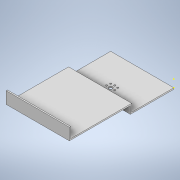
# Autodesk Inventor part: Single Sided board
Saved by Autodesk Inventor 2020.3 (Build 243373010, 373A)
## iProperties
Created: 2020-09-26
Part Number: Single Sided board
Material: Generic
Document SubType Name: Modeling
Designer: Owner
Density: 1 g/cm^3
Appearance: Default
Author: Owner
Autodesk Inventor part; units mm, degrees
ref_plane "YZ Plane" through (0, 0, 0) normal (1, 0, 0) x (0, 1, 0)
ref_plane "XZ Plane" through (0, 0, 0) normal (0, 1, 0) x (-1, 0, 0)
ref_plane "XY Plane" through (0, 0, 0) normal (0, 0, 1) x (1, 0, 0)
sketch "Sketch1" plane through (0, 0, 0) normal (0, 1, 0) x (-1, 0, 0)
  line L0 (0, 0) -> (152.4, 0)
  line L1 (152.4, 0) -> (152.4, 252.095)
  line L2 (152.4, 252.095) -> (0, 252.095)
  line L3 (0, 252.095) -> (0, 0)
  circle A0 centre (76.2, 76.2) radius 50.8
  circle A1 centre (76.2, 76.2) radius 4.5
  dimension "d0" = 152.4
  dimension "d1" = 252.095
  dimension "d2" = 101.6
  dimension "d3" = 9
  constraints: 8 end point, 2 centre point, 2 parallel, 1 coincident, 1 horizontal, 1 perpendicular
  measures "d0" distance of L2.end L1.end
  measures "d1" distance of L1.end L0.end
  measures "d2" diameter of A0
  measures "d3" diameter of A1
extrude "Extrusion1" add sketch "Sketch1" against normal blind 3.175 contours L3 L2 L1 L0 | A0
sketch "Sketch2" plane through (0, 0, 0) normal (0, 1, 0) x (1, 0, 0)
  line L0 (0, -252.095) -> (-152.4, -252.095) projected
  line L1 (-152.4, -252.095) -> (-152.4, 0) projected
  line L2 (0, -252.095) -> (-152.4, -252.095)
  line L3 (-152.4, -252.095) -> (-152.4, -248.92)
  line L4 (-152.4, -248.92) -> (0, -248.92)
  line L5 (0, -248.92) -> (0, -252.095)
  point P0 (0, 0)
  dimension "d6" = 3.175
  constraints: 8 end point, 2 parallel, 1 horizontal, 1 perpendicular, 1 point on line
  measures "d6" distance of L2.end L3.end
extrude "Extrusion2" add sketch "Sketch2" along normal blind 25.4
sketch "Sketch3" plane through (0, 0, 0) normal (0, 1, 0) x (1, 0, 0)
  circle A0 centre (-66.421, -76.2) radius 2
  circle A1 centre (-85.979, -76.2) radius 2
  circle A2 centre (-76.2, -66.421) radius 2
  circle A3 centre (-76.2, -85.979) radius 2
  point P0 (0, 0)
  dimension "d9" = 4
  dimension "d10" = 4
  dimension "d11" = 4
  dimension "d12" = 4
  constraints: 4 centre point
  measures "d9" diameter of A0
  measures "d10" diameter of A1
  measures "d11" diameter of A2
  measures "d12" diameter of A3
extrude "Extrusion3" cut sketch "Sketch3" against normal blind 25.4
sketch "Sketch4" plane through (0, 0, 0) normal (0, 1, 0) x (1, 0, 0)
  circle A0 centre (-76.2, -85.979) radius 2 projected
  circle A1 centre (-76.2, -85.979) radius 2
  circle A2 centre (-76.2, -76.2) radius 4.5 projected
  circle A3 centre (-76.2, -76.2) radius 4.5
  circle A4 centre (-83.1148, -83.1148) radius 2
  circle A5 centre (-76.2, -76.2) radius 4.5
  circle A6 centre (-85.979, -76.2) radius 2
  circle A7 centre (-76.2, -76.2) radius 4.5
  circle A8 centre (-83.1148, -69.2852) radius 2
  circle A9 centre (-76.2, -76.2) radius 4.5
  circle A10 centre (-76.2, -66.421) radius 2
  circle A11 centre (-76.2, -76.2) radius 4.5
  circle A12 centre (-69.2852, -69.2852) radius 2
  circle A13 centre (-76.2, -76.2) radius 4.5
  circle A14 centre (-66.421, -76.2) radius 2
  circle A15 centre (-76.2, -76.2) radius 4.5
  circle A16 centre (-69.2852, -83.1148) radius 2
  circle A17 centre (-76.2, -76.2) radius 4.5
  point P0 (0, 0)
  dimension "d17" = 360
  constraints: 18 coincident, 16 centre point, 47 other
extrude "Extrusion4" cut sketch "Sketch4" against normal blind 25.4 contours A4 | A8 | A12 | A16
sketch "Sketch5" plane through (0, 0, 0) normal (0, 1, 0) x (1, 0, 0)
  point P0 (0, 0)
sketch "Sketch6" plane through (0, 0, 0) normal (0, 1, 0) x (1, 0, 0)
  point P0 (0, 0)
sketch "Sketch7" plane through (0, -3.175, 0) normal (0, -1, 0) x (1, 0, 0)
  circle A0 centre (-83.1148, 83.1148) radius 2 projected
  circle A1 centre (-83.1148, 83.1148) radius 2.8284
  circle A2 centre (-83.1148, 69.2852) radius 2 projected
  circle A3 centre (-83.1148, 69.2852) radius 2.8284
  circle A4 centre (-69.2852, 69.2852) radius 2 projected
  circle A5 centre (-69.2852, 69.2852) radius 2.9799
  circle A6 centre (-69.2852, 83.1148) radius 29.4992
  circle A7 centre (-69.2852, 83.1148) radius 2 projected
  circle A8 centre (-69.2852, 83.1148) radius 3.4641
  point P0 (0, 0)
  constraints: 5 centre point, 4 coincident
extrude "Extrusion5" add sketch "Sketch7" against normal blind 3.175 contours A0 | A1 | A2 | A3 | A4 | A5 | A7 | A8
sketch "Sketch8" plane through (0, 0, 0) normal (0, 1, 0) x (1, 0, 0)
  circle A0 centre (-76.2, -76.2) radius 4.5 projected
  circle A1 centre (-76.2, -76.2) radius 4.5
  circle A2 centre (-64.2, -76.2) radius 2
  circle A3 centre (-76.2, -76.2) radius 4.5
  circle A4 centre (-76.2, -76.2) radius 4.5
  circle A5 centre (-76.2, -76.2) radius 4.5
  circle A6 centre (-76.2, -76.2) radius 4.5
  circle A7 centre (-76.2, -76.2) radius 4.5
  circle A8 centre (-76.2, -76.2) radius 4.5
  circle A9 centre (-76.2, -76.2) radius 4.5
  circle A10 centre (-67.7147, -84.6853) radius 2
  circle A11 centre (-84.6853, -84.6853) radius 2
  circle A12 centre (-84.6853, -67.7147) radius 2
  circle A13 centre (-67.7147, -67.7147) radius 2
  point P0 (0, 0)
  point P1 (-76.2, -64.2)
  point P2 (-88.2, -76.2)
  point P3 (-76.2, -88.2)
  dimension "d23" = 4
  dimension "d26" = 360
  dimension "d28" = 4
  dimension "d29" = 4
  dimension "d30" = 4
  dimension "d31" = 4
  constraints: 13 centre point, 5 coincident, 25 other
  measures "d23" diameter of A2
  measures "d28" diameter of A10
  measures "d29" diameter of A11
  measures "d30" diameter of A12
  measures "d31" diameter of A13
extrude "Extrusion6" cut sketch "Sketch8" against normal blind 25.4 contours A10 | A11 | A12 | A13
sketch "Sketch9" plane through (0, 25.4, 0) normal (0, 1, 0) x (1, 0, 0)
  line L0 (0, -248.92) -> (0, 0) projected
  line L1 (-163.9684, -278.6073) -> (0, -278.6073)
  line L2 (0, -278.6073) -> (0, -205.6552)
  line L3 (0, -205.6552) -> (-163.9684, -205.6552)
  line L4 (-163.9684, -205.6552) -> (-163.9684, -278.6073)
  constraints: 8 end point, 2 parallel, 1 horizontal, 1 perpendicular, 1 point on line
extrude "Extrusion7" cut sketch "Sketch9" against normal blind 25.4
sketch "Sketch10" plane through (0, 0, 0) normal (0, 1, 0) x (1, 0, 0)
  line L0 (-152.4, -252.095) -> (-152.4, 0) projected
  line L1 (0, -101.6) -> (-152.4, -101.6)
  line L2 (-152.4, -101.6) -> (-152.4, -252.095)
  line L3 (-152.4, -252.095) -> (0, -252.095)
  line L4 (0, -252.095) -> (0, -101.6)
  point P0 (0, 0)
  constraints: 8 end point, 2 parallel, 1 horizontal, 1 perpendicular
extrude "Extrusion8" add sketch "Sketch10" along normal blind 18.288
sketch "Sketch11" plane through (0, 18.288, 0) normal (0, 1, 0) x (1, 0, 0)
  point P0 (0, 0)
sketch "Sketch12" plane through (0, 18.288, 0) normal (0, 1, 0) x (1, 0, 0)
  line L0 (0, -252.095) -> (-152.4, -252.095) projected
  line L1 (-152.4, -252.095) -> (0, -252.095)
  line L2 (0, -252.095) -> (0, -248.92)
  line L3 (0, -248.92) -> (-152.4, -248.92)
  line L4 (-152.4, -248.92) -> (-152.4, -252.095)
  point P0 (0, 0)
  dimension "d38" = 3.175
  constraints: 8 end point, 2 parallel, 1 horizontal, 1 perpendicular
  measures "d38" distance of L2.end L1.end
extrude "Extrusion9" add sketch "Sketch12" along normal blind 25.4
sketch "Sketch13" plane through (0, -3.175, 252.095) normal (1, 0, 0) x (0, 0, -1)
  line L0 (150.495, 3.175) -> (150.495, 21.463) projected
  line L1 (0, 0) -> (0, 46.863) projected
  line L2 (150.495, 21.463) -> (0, 21.463)
  line L3 (0, 21.463) -> (0, 18.288)
  line L4 (0, 18.288) -> (150.495, 18.288)
  line L5 (150.495, 18.288) -> (150.495, 21.463)
  line L6 (252.095, 0) -> (0, 0) projected
  line L7 (150.495, 21.463) -> (147.32, 21.463)
  line L8 (147.32, 21.463) -> (147.32, 0)
  line L9 (147.32, 0) -> (150.495, 0)
  line L10 (150.495, 0) -> (150.495, 21.463)
  line L11 (0, 18.288) -> (147.32, 18.288)
  line L12 (147.32, 18.288) -> (147.32, 0)
  line L13 (147.32, 0) -> (0, 0)
  line L14 (0, 0) -> (0, 18.288)
  point P0 (252.095, 3.175)
  dimension "d41" = 3.175
  dimension "d42" = 3.175
  constraints: 24 end point, 6 parallel, 3 horizontal, 3 perpendicular, 2 point on line
  measures "d41" distance of L3.end L2.end
  measures "d42" distance of L9.end L8.end
extrude "Extrusion10" cut sketch "Sketch13" against normal blind 254 contours L8 L6 L1 L4
body "Solid1"
